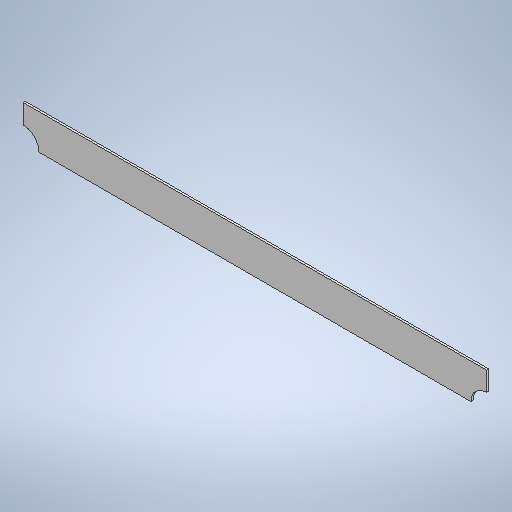
# Autodesk Inventor part: MSC 0562 rib cone
Saved by Autodesk Inventor 2025 (Build 290162010, 162A)
## iProperties
Created: 2024-06-26
Part Number: MSC 0562 rib cone
Material: Stainless Steel
Document SubType Name: Sheet Metal
Designer: pokla
Density: 8 g/cm^3
Sheet Metal Rule: AISI304 3mm Die 32
Appearance: Default
Author: pokla
Autodesk Inventor part; units mm, degrees
ref_plane "YZ Plane" through (0, 0, 0) normal (1, 0, 0) x (0, 1, 0)
ref_plane "XZ Plane" through (0, 0, 0) normal (0, 1, 0) x (-1, 0, 0)
ref_plane "XY Plane" through (0, 0, 0) normal (0, 0, 1) x (1, 0, 0)
sketch "Sketch2" plane through (0, 0, 0) normal (0, 1, 0) x (-1, 0, 0)
  line L0 (330, 50) -> (-330, 50)
  line L1 (-330, 50) -> (-330, 0)
  line L2 (-330, 0) -> (330, 0)
  line L3 (330, 0) -> (330, 50)
  circle A0 centre (-330, 0) radius 22.5
  circle A1 centre (330, 0) radius 22.5
  point P0 (0, 0)
  point P1 (0, 0)
  point P2 (-330, 22.5)
  point P3 (-307.5, 0)
  point P4 (307.5, 0)
  point P5 (330, 22.5)
  dimension "d18" = 660
  dimension "d19" = 50
  dimension "d20" = 45
  measures "d18" distance of L2.end L1.end
  measures "d19" distance of L1.end L0.end
  measures "d20" diameter of A0
extrude "Plate2" add sketch "Sketch2" along normal blind 3 contours L3 A1 L2 A0 L1 L0
equation "\"d21\" = Thickness"
equation "\"BendReliefWidth\" = Thickness"
equation "\"BendReliefDepth\" = 0.5 * Thickness"
equation "\"CornerReliefSize\" = 4 * Thickness"
equation "\"MinimumRemnant\" = 2 * Thickness"
equation "\"TransitionRadius\" = BendRadius"
equation "\"JacobiRadiusSize\" = BendRadius"
equation "\"GapSize\" = Thickness"
equation "\"Thickness\" = 3"
equation "\"BendRadius\" = 5"
body "Solid2"
